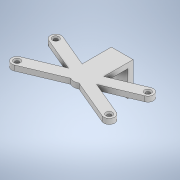
# Autodesk Inventor part: HolderSR04
Saved by Autodesk Inventor 2021 (Build 250183000, 183)
## iProperties
Created: 2021-06-08
Part Number: HolderSR04
Material: Generisch
Document SubType Name: Modeling
Designer: User
Density: 1 g/cm^3
Appearance: Vorgabe
Author: User
Autodesk Inventor part; units mm, degrees
ref_plane "YZ Plane" through (0, 0, 0) normal (1, 0, 0) x (0, 1, 0)
ref_plane "XZ Plane" through (0, 0, 0) normal (0, 1, 0) x (-1, 0, 0)
derived "HC-SR04.ipt"
sketch "Skizze1" plane through (-22.6, 0, 10.3) normal (0, -1, 0) x (1, 0, 0)
  line L0 (0, 0) -> (45.2, 0) projected
  line L1 (45.2, 0) -> (45.2, -20.6) projected
  line L2 (45.2, -20.6) -> (0, -20.6) projected
  line L3 (0, -20.6) -> (0, 0) projected
  circle A0 centre (1.4, -1.4) radius 1 projected
  circle A1 centre (43.8, -19.2) radius 1 projected
  line L4 (27.68, -2) -> (27.68, -0.5) projected
  line L5 (27.18, -2.5) -> (27.68, -2) projected
  line L6 (25.64, -2.5) -> (27.18, -2.5) projected
  line L7 (23.1, -2.5) -> (24.64, -2.5) projected
  line L8 (20.56, -2.5) -> (22.1, -2.5) projected
  line L9 (18.02, -2.5) -> (19.56, -2.5) projected
  line L10 (17.52, -2) -> (18.02, -2.5) projected
  line L11 (17.52, -0.5) -> (17.52, -2) projected
  line L12 (18.02, 0) -> (17.52, -0.5) projected
  line L13 (43.8, -19.2) -> (1.4, -1.4) construction
  line L14 (1.4, -1.4) -> (1.4, -19.2) construction
  line L15 (1.4, -19.2) -> (43.8, -19.2) construction
  line L16 (43.8, -1.4) -> (1.4, -1.4) construction
  line L17 (43.8, -1.4) -> (43.8, -19.2) construction
  circle A2 centre (43.8, -1.4) radius 0.9
  circle A3 centre (1.4, -19.2) radius 0.9
  circle A4 centre (43.8, -19.2) radius 0.9
  circle A5 centre (1.4, -1.4) radius 0.9
  line L18 (20.6886, -6.7862) -> (2.3677, 0.9051)
  line L19 (0.4323, -3.7051) -> (18.7532, -11.3964)
  line L20 (18.7532, -9.2036) -> (0.4323, -16.8949)
  line L21 (2.3677, -21.5051) -> (20.6886, -13.8138)
  line L22 (24.5114, -13.8138) -> (42.8323, -21.5051)
  line L23 (44.7677, -16.8949) -> (26.4468, -9.2036)
  line L24 (26.4468, -11.3964) -> (44.7677, -3.7051)
  line L25 (44.0903, -2.0915) -> (43.5097, -0.7085) construction
  line L26 (43.8, -1.4) -> (1.4, -19.2) construction
  circle A6 centre (22.6, -10.3) radius 4
  line L27 (42.8323, 0.9051) -> (24.5114, -6.7862)
  circle A7 centre (43.8, -1.4) radius 2.5
  circle A8 centre (43.8, -19.2) radius 2.5
  circle A9 centre (1.4, -19.2) radius 2.5
  circle A10 centre (1.4, -1.4) radius 2.5
  circle A11 centre (43.8, -1.4) radius 1.5 construction
  circle A12 centre (43.8, -19.2) radius 1.5 construction
  circle A13 centre (1.4, -19.2) radius 1.5 construction
  circle A14 centre (1.4, -1.4) radius 1.5 construction
  line L28 (27.6, -15.1104) -> (27.6, -28.6)
  line L29 (27.6, -28.6) -> (17.6, -28.6)
  line L30 (17.6, -28.6) -> (17.6, -15.1104)
  line L31 (22.6, -10.3) -> (22.6, -28.6) construction
  line L32 (27.6, -26.2) -> (17.6, -26.2)
  point P0 (29.0585, -10.3)
  point P1 (41.7288, 0)
  point P2 (40.6763, 0)
  point P3 (16.1415, -10.3)
  dimension "d3" = 8
  dimension "d1" = 1.8
  dimension "d5" = 5
  dimension "d6" = 5
  dimension "d7" = 5
  dimension "d8" = 5
  dimension "d9" = 5
  dimension "d10" = 5
  dimension "d11" = 5
  dimension "d12" = 5
  dimension "d13" = 3
  dimension "d14" = 10
  dimension "d15" = 8
  dimension "d16" = 2.4
  constraints: 40 end point, 12 centre point, 12 coincident, 8 point on circle, 7 perpendicular, 6 equal radius, 4 parallel, 4 point on line, 4 vertical, 3 midpoint, 14 other
  measures "d1" diameter of A2
  measures "d5" distance between parallel lines of L24 L27
  measures "d6" distance between parallel lines of L22 L23
  measures "d7" distance between parallel lines of L21 L20
  measures "d8" distance between parallel lines of L18 L19
  measures "d9" diameter of A7
  measures "d10" diameter of A8
  measures "d11" diameter of A9
  measures "d12" diameter of A10
  measures "d13" diameter of A11
  measures "d14" distance of L28.end L29.end
  measures "d15" distance between parallel lines of L2 L29
  measures "d16" distance between parallel lines of L29 L32
extrude "Extrusion1" add sketch "Skizze1" along normal blind 2.4 contours L3 A10 L0 | L0 A10 L3 | A10 L18 L0 | L0 L18 A6 L20 L19 A10 | A9 L2 L3 | L3 L2 A9 | A6 | L20 L19 A6 L21 L2 A9 | A9 L2 L21 | L20 A6 L19 | L27 A7 L0 | L0 A7 L24 L23 A6 L27 | A7 L1 L0 | L0 L1 A7 | L23 L24 A6 | L30 L21 A6 L22 L28 L2 | L2 L28 L32 L30 | L23 A8 L2 L22 A6 L24 | L32 L28 L29 L30 | A8 L1 L2 | L2 A8 L22 | A8 L2 L1 | A0 | A1 | A2 | A3 | A4 | A5
sketch "Skizze3" plane through (-5, -2.4, -18.3) normal (0, -1, 0) x (1, 0, 0)
  line L0 (10, 0) -> (10, 13.4896) projected
  line L1 (0, 13.4896) -> (0, 0) projected
  line L2 (0, 0) -> (10, 0) projected
  line L3 (10, 2.4) -> (0, 2.4) projected
  point P0 (5, 18.3)
extrude "Extrusion2" add sketch "Skizze3" along normal blind 12
ref_plane "Arbeitsebene1" through (-5, 2.4, -18.3) normal (0, 1, 0) x (1, 0, 0)
extrude "Extrusion3" cut sketch "Skizze1" along normal through all contours A2 | A3 | A4 | A5
sketch "Skizze4" plane through (-5, -2.4, -15.9) normal (0, 0, 1) x (1, 0, 0)
  circle A0 centre (2.8852, -3.4622) radius 2.1
  circle A1 centre (7.1148, -8.5378) radius 2.1
  line L0 (-15.2323, 0) -> (0, 0) construction
  line L1 (0, 0) -> (10, -12) construction
  point P0 (5, 2.4)
  dimension "d25" = 15.6205
  dimension "d27" = 4.5068
  dimension "d28" = 4.2
  dimension "d30" = 4.5068
  constraints: 2 centre point, 2 end point, 2 point on line, 1 coincident, 1 equal radius
  measures "d25" distance of L0.end L1.end
  measures "d27" distance of L0.end A0.centre
  measures "d28" diameter of A1
  measures "d30" distance of A1.centre L1.end
extrude "Extrusion4" cut sketch "Skizze4" against normal blind 12
chamfer "Fase1" distance 0.6 angle 45 4 edges at (20.3, 0, 8.9) (20.3, 0, -8.9) (-22.1, 0, -8.9) (-22.1, 0, 8.9)
equation "\"d6\" = d5"
equation "\"d7\" = d5"
equation "\"d8\" = d5"
equation "\"d10\" = d9"
equation "\"d11\" = d10"
equation "\"d12\" = d9"
equation "\"d27\" = d30"
equation "\"d30\" = 0.333333 * d25 - 0.166667 * d28"
equation "\"d26\" = 0.119048 * d25"
